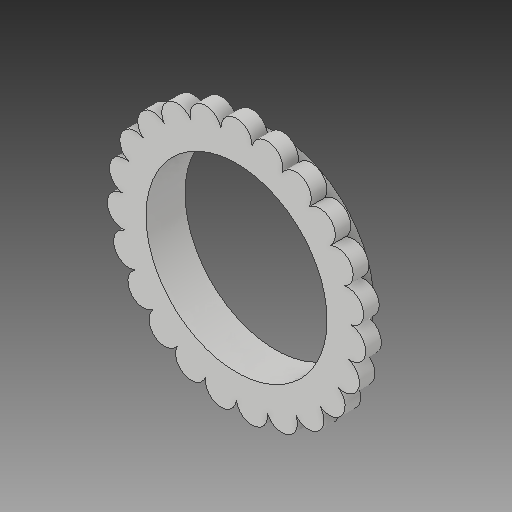
# Autodesk Inventor part: 20_Lens_holder_clamp
Saved by Autodesk Inventor 2019 (Build 230136000, 136)
## iProperties
Created: 2019-10-23
Part Number: 20_Lens_holder_clamp
Material: Generic
Document SubType Name: Modeling
Designer: marsikovabarbora
Density: 1 g/cm^3
Appearance: Default
Author: marsikovabarbora
Autodesk Inventor part; units mm, degrees
ref_plane "YZ Plane" through (0, 0, 0) normal (1, 0, 0) x (0, 1, 0)
ref_plane "XZ Plane" through (0, 0, 0) normal (0, 1, 0) x (-1, 0, 0)
ref_plane "XY Plane" through (0, 0, 0) normal (0, 0, 1) x (1, 0, 0)
sketch "Sketch1" plane through (0, 0, 0) normal (0, 0, 1) x (1, 0, 0)
  circle A0 centre (0, 0) radius 12.85
  line L0 (16.8, 24.9006) -> (-16.8, 24.9006) projected
  line L1 (-16.8, 24.9006) -> (-16.8, 21.2406) projected
  line L2 (-16.8, 21.2406) -> (-21.2406, 16.8) projected
  line L3 (-21.2406, 16.8) -> (-24.9006, 16.8) projected
  line L4 (-24.9006, 16.8) -> (-24.9006, -16.8) projected
  line L5 (-24.9006, -16.8) -> (-21.2406, -16.8) projected
  line L6 (-21.2406, -16.8) -> (-16.8, -21.2406) projected
  line L7 (-16.8, -21.2406) -> (-16.8, -24.9006) projected
  line L8 (-16.8, -24.9006) -> (16.8, -24.9006) projected
  line L9 (16.8, -24.9006) -> (16.8, -21.2406) projected
  line L10 (16.8, -21.2406) -> (21.2406, -16.8) projected
  line L11 (21.2406, -16.8) -> (24.9006, -16.8) projected
  line L12 (24.9006, -16.8) -> (24.9006, 16.8) projected
  line L13 (24.9006, 16.8) -> (21.2406, 16.8) projected
  line L14 (21.2406, 16.8) -> (16.8, 21.2406) projected
  line L15 (16.8, 21.2406) -> (16.8, 24.9006) projected
  circle A1 centre (0, 0) radius 12.6
  circle A2 centre (0, 0) radius 11.6
  point P0 (0, 0)
  dimension "d0" = 0.25
  dimension "d1" = 1
  dimension "d11" = 25.7
  constraints: 3 centre point
  measures "d0" radial gap between concentric circles of A0 A1
  measures "d1" radial gap between concentric circles of A1 A2
  measures "d11" diameter of A0
ref_plane "Work Plane1" through (-13.5, -13.5, -4) normal (0, 0, 1) x (1, 0, 0)
extrude "Extrusion1" add sketch "Sketch1" against normal blind 3 contours A1
sketch "Sketch2" plane through (0, 0, 0) normal (0, 0, 1) x (1, 0, 0)
  circle A0 centre (0, 0) radius 11.6 projected
  circle A1 centre (0, 0) radius 14.6
  line L0 (0, -21.12) -> (0, 23.12) construction
  arc A2 (1.9953, 14.463) -> (-1.9953, 14.463) centre (0, 14.6) ccw
  point P0 (0, 0)
  dimension "d4" = 3
  dimension "d5" = 2
  constraints: 5 point on circle, 2 centre point, 1 point on line
  measures "d4" radial gap between concentric circles of A0 A1
  measures "d5" radius of A2
extrude "Extrusion2" add sketch "Sketch2" along normal blind 2
pattern_circular "Circular Pattern1" count 23 over 360 about axis through (0, 0, -10) along (0, 0, 1) of "Extrusion2"
body "Solid1"
